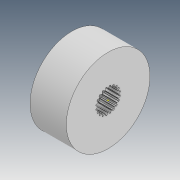
# Autodesk Inventor part: roda certa 3.0
Saved by Autodesk Inventor 2021 (Build 250183000, 183)
## iProperties
Created: 2020-10-21
Part Number: roda certa 3.0
Material: Genérico
Document SubType Name: Modeling
Designer: evert
Density: 1 g/cm^3
Appearance: Padrão
Author: evert
Autodesk Inventor part; units mm, degrees
ref_plane "YZ Plane" through (0, 0, 0) normal (1, 0, 0) x (0, 1, 0)
ref_plane "XZ Plane" through (0, 0, 0) normal (0, 1, 0) x (-1, 0, 0)
ref_plane "XY Plane" through (0, 0, 0) normal (0, 0, 1) x (1, 0, 0)
sketch "Esboço2" plane through (0, 0, 0) normal (0, 0, 1) x (1, 0, 0)
  line L0 (0, 0) -> (9.5, 0)
  line L1 (9.5, 0) -> (9.5, 9.8)
  line L2 (9.5, 9.8) -> (0, 9.8)
  line L3 (0, 9.8) -> (0, 0)
  line L4 (9.5, 0) -> (1, 0)
  line L5 (9.5, 0) -> (0.5, 0)
  line L6 (0, 0) -> (1, 0)
  line L7 (1, 0) -> (1, 9.8)
  dimension "d0" = 9.5
  dimension "d1" = 9.8
  dimension "d71" = 8.5
  dimension "d72" = 9
  constraints: 16 end point, 3 point on line, 2 parallel, 2 perpendicular, 1 collinear, 1 horizontal
  measures "d0" distance of L1.end L2.end
  measures "d1" distance of L0.end L1.end
  measures "d71" distance of L0.end L4.end
  measures "d72" distance of L0.end L5.end
revolve "Revolução1" add sketch "Esboço2" angle 360 about axis through (0, 0, 0) along (1, 0, 0) contours L7 L2 L1 L0
sketch "Esboço12" plane through (9.5, 0, 0) normal (1, 0, 0) x (0, 0, -1)
  point P0 (0, 0)
sketch "Esboço13" plane through (1, 0, 0) normal (-1, 0, 0) x (0, 0, 1)
  circle A0 centre (0, 0) radius 1.75
  dimension "d73" = 3.5
  constraints: 1 centre point, 1 coincident
  measures "d73" diameter of A0
extrude "Extrusão6" cut sketch "Esboço13" against normal blind 3.85
sketch "Esboço14" plane through (1, 0, 0) normal (-1, 0, 0) x (0, 0, 1)
  circle A0 centre (0, 0) radius 1.75 projected
  circle A1 centre (0, 0) radius 4.5
  dimension "d76" = 9
  constraints: 1 centre point, 1 coincident
  measures "d76" diameter of A1
extrude "Extrusão7" cut sketch "Esboço14" against normal blind 1
sketch "Esboço15" plane through (9.5, 0, 0) normal (1, 0, 0) x (0, 0, -1)
  circle A0 centre (0, 0) radius 2.5
  circle A1 centre (0, 0) radius 1.75 projected
  circle A2 centre (0, 0) radius 2.9
  line L0 (2.5, 0) -> (2.5, 0.05)
  line L1 (2.5, 0) -> (2.4995, -0.05)
  line L2 (2.4995, -0.05) -> (2.8824, -0.3191)
  line L3 (2.5, 0.05) -> (2.8824, 0.3191)
  line L4 (2.8824, 0.3191) -> (2.8765, 0.3688)
  line L5 (2.8824, -0.3191) -> (2.8824, -0.3191)
  line L6 (2.8824, -0.3191) -> (2.8824, -0.3191)
  line L7 (2.8824, -0.3191) -> (2.8824, -0.3191)
  line L8 (2.8824, -0.3191) -> (2.8824, -0.3191)
  line L9 (2.8824, -0.3191) -> (2.8824, -0.3191)
  line L10 (2.8795, -0.3439) -> (2.8795, -0.3439)
  line L11 (2.8824, -0.3191) -> (2.8824, -0.3191)
  line L12 (2.3622, 0.8201) -> (2.6427, 1.1942)
  line L13 (2.6427, 1.1942) -> (2.6217, 1.2396)
  line L14 (2.3776, 0.7725) -> (2.3622, 0.8201)
  line L15 (2.3776, 0.7725) -> (2.3926, 0.7248)
  line L16 (2.3926, 0.7248) -> (2.8399, 0.5872)
  circle A3 centre (0, 0) radius 2.9
  line L17 (1.9932, 1.5099) -> (2.1443, 1.9524)
  line L18 (2.1443, 1.9524) -> (2.1104, 1.9891)
  line L19 (2.0225, 1.4695) -> (1.9932, 1.5099)
  line L20 (2.0225, 1.4695) -> (2.0515, 1.4287)
  line L21 (2.0515, 1.4287) -> (2.5195, 1.4361)
  circle A4 centre (0, 0) radius 2.9
  line L22 (1.429, 2.0519) -> (1.4361, 2.5195)
  line L23 (1.4361, 2.5195) -> (1.3924, 2.5439)
  line L24 (1.4695, 2.0225) -> (1.429, 2.0519)
  line L25 (1.4695, 2.0225) -> (1.5096, 1.9928)
  line L26 (1.5096, 1.9928) -> (1.9524, 2.1443)
  circle A5 centre (0, 0) radius 2.9
  line L27 (0.725, 2.3931) -> (0.5872, 2.8399)
  line L28 (0.5872, 2.8399) -> (0.5382, 2.8496)
  line L29 (0.7725, 2.3776) -> (0.725, 2.3931)
  line L30 (0.7725, 2.3776) -> (0.8199, 2.3617)
  line L31 (0.8199, 2.3617) -> (1.1942, 2.6427)
  circle A6 centre (0, 0) radius 2.9
  line L32 (-0.05, 2.5) -> (-0.3191, 2.8824)
  line L33 (-0.3191, 2.8824) -> (-0.3688, 2.8765)
  line L34 (0, 2.5) -> (-0.05, 2.5)
  line L35 (0, 2.5) -> (0.05, 2.4995)
  line L36 (0.05, 2.4995) -> (0.3191, 2.8824)
  circle A7 centre (0, 0) radius 2.9
  line L37 (-0.8201, 2.3622) -> (-1.1942, 2.6427)
  line L38 (-1.1942, 2.6427) -> (-1.2396, 2.6217)
  line L39 (-0.7725, 2.3776) -> (-0.8201, 2.3622)
  line L40 (-0.7725, 2.3776) -> (-0.7248, 2.3926)
  line L41 (-0.7248, 2.3926) -> (-0.5872, 2.8399)
  circle A8 centre (0, 0) radius 2.9
  line L42 (-1.5099, 1.9932) -> (-1.9524, 2.1443)
  line L43 (-1.9524, 2.1443) -> (-1.9891, 2.1104)
  line L44 (-1.4695, 2.0225) -> (-1.5099, 1.9932)
  line L45 (-1.4695, 2.0225) -> (-1.4287, 2.0515)
  line L46 (-1.4287, 2.0515) -> (-1.4361, 2.5195)
  circle A9 centre (0, 0) radius 2.9
  line L47 (-2.0519, 1.429) -> (-2.5195, 1.4361)
  line L48 (-2.5195, 1.4361) -> (-2.5439, 1.3924)
  line L49 (-2.0225, 1.4695) -> (-2.0519, 1.429)
  line L50 (-2.0225, 1.4695) -> (-1.9928, 1.5096)
  line L51 (-1.9928, 1.5096) -> (-2.1443, 1.9524)
  circle A10 centre (0, 0) radius 2.9
  line L52 (-2.3931, 0.725) -> (-2.8399, 0.5872)
  line L53 (-2.8399, 0.5872) -> (-2.8496, 0.5382)
  line L54 (-2.3776, 0.7725) -> (-2.3931, 0.725)
  line L55 (-2.3776, 0.7725) -> (-2.3617, 0.8199)
  line L56 (-2.3617, 0.8199) -> (-2.6427, 1.1942)
  circle A11 centre (0, 0) radius 2.9
  line L57 (-2.5, -0.05) -> (-2.8824, -0.3191)
  line L58 (-2.8824, -0.3191) -> (-2.8765, -0.3688)
  line L59 (-2.5, 0) -> (-2.5, -0.05)
  line L60 (-2.5, 0) -> (-2.4995, 0.05)
  line L61 (-2.4995, 0.05) -> (-2.8824, 0.3191)
  circle A12 centre (0, 0) radius 2.9
  line L62 (-2.3622, -0.8201) -> (-2.6427, -1.1942)
  line L63 (-2.6427, -1.1942) -> (-2.6217, -1.2396)
  line L64 (-2.3776, -0.7725) -> (-2.3622, -0.8201)
  line L65 (-2.3776, -0.7725) -> (-2.3926, -0.7248)
  line L66 (-2.3926, -0.7248) -> (-2.8399, -0.5872)
  circle A13 centre (0, 0) radius 2.9
  line L67 (-1.9932, -1.5099) -> (-2.1443, -1.9524)
  line L68 (-2.1443, -1.9524) -> (-2.1104, -1.9891)
  line L69 (-2.0225, -1.4695) -> (-1.9932, -1.5099)
  line L70 (-2.0225, -1.4695) -> (-2.0515, -1.4287)
  line L71 (-2.0515, -1.4287) -> (-2.5195, -1.4361)
  circle A14 centre (0, 0) radius 2.9
  line L72 (-1.429, -2.0519) -> (-1.4361, -2.5195)
  line L73 (-1.4361, -2.5195) -> (-1.3924, -2.5439)
  line L74 (-1.4695, -2.0225) -> (-1.429, -2.0519)
  line L75 (-1.4695, -2.0225) -> (-1.5096, -1.9928)
  line L76 (-1.5096, -1.9928) -> (-1.9524, -2.1443)
  circle A15 centre (0, 0) radius 2.9
  line L77 (-0.725, -2.3931) -> (-0.5872, -2.8399)
  line L78 (-0.5872, -2.8399) -> (-0.5382, -2.8496)
  line L79 (-0.7725, -2.3776) -> (-0.725, -2.3931)
  line L80 (-0.7725, -2.3776) -> (-0.8199, -2.3617)
  line L81 (-0.8199, -2.3617) -> (-1.1942, -2.6427)
  circle A16 centre (0, 0) radius 2.9
  line L82 (0.05, -2.5) -> (0.3191, -2.8824)
  line L83 (0.3191, -2.8824) -> (0.3688, -2.8765)
  line L84 (0, -2.5) -> (0.05, -2.5)
  line L85 (0, -2.5) -> (-0.05, -2.4995)
  line L86 (-0.05, -2.4995) -> (-0.3191, -2.8824)
  circle A17 centre (0, 0) radius 2.9
  line L87 (0.8201, -2.3622) -> (1.1942, -2.6427)
  line L88 (1.1942, -2.6427) -> (1.2396, -2.6217)
  line L89 (0.7725, -2.3776) -> (0.8201, -2.3622)
  line L90 (0.7725, -2.3776) -> (0.7248, -2.3926)
  line L91 (0.7248, -2.3926) -> (0.5872, -2.8399)
  circle A18 centre (0, 0) radius 2.9
  line L92 (1.5099, -1.9932) -> (1.9524, -2.1443)
  line L93 (1.9524, -2.1443) -> (1.9891, -2.1104)
  line L94 (1.4695, -2.0225) -> (1.5099, -1.9932)
  line L95 (1.4695, -2.0225) -> (1.4287, -2.0515)
  line L96 (1.4287, -2.0515) -> (1.4361, -2.5195)
  circle A19 centre (0, 0) radius 2.9
  line L97 (2.0519, -1.429) -> (2.5195, -1.4361)
  line L98 (2.5195, -1.4361) -> (2.5439, -1.3924)
  line L99 (2.0225, -1.4695) -> (2.0519, -1.429)
  line L100 (2.0225, -1.4695) -> (1.9928, -1.5096)
  line L101 (1.9928, -1.5096) -> (2.1443, -1.9524)
  circle A20 centre (0, 0) radius 2.9
  line L102 (2.3931, -0.725) -> (2.8399, -0.5872)
  line L103 (2.8399, -0.5872) -> (2.8496, -0.5382)
  line L104 (2.3776, -0.7725) -> (2.3931, -0.725)
  line L105 (2.3776, -0.7725) -> (2.3617, -0.8199)
  line L106 (2.3617, -0.8199) -> (2.6427, -1.1942)
  circle A21 centre (0, 0) radius 2.9
  point P0 (2.8399, 0.5872)
  point P1 (2.8399, 0.5872)
  point P2 (2.8399, 0.5872)
  point P3 (2.8399, 0.5872)
  point P4 (2.8399, 0.5872)
  point P5 (2.8449, 0.5627)
  point P6 (2.8449, 0.5627)
  point P7 (2.8399, 0.5872)
  point P8 (2.5195, 1.4361)
  point P9 (2.5195, 1.4361)
  point P10 (2.5195, 1.4361)
  point P11 (2.5195, 1.4361)
  point P12 (2.5195, 1.4361)
  point P13 (2.5318, 1.4143)
  point P14 (2.5318, 1.4143)
  point P15 (2.5195, 1.4361)
  point P16 (1.9524, 2.1443)
  point P17 (1.9524, 2.1443)
  point P18 (1.9524, 2.1443)
  point P19 (1.9524, 2.1443)
  point P20 (1.9524, 2.1443)
  point P21 (1.9708, 2.1274)
  point P22 (1.9708, 2.1274)
  point P23 (1.9524, 2.1443)
  point P24 (1.1942, 2.6427)
  point P25 (1.1942, 2.6427)
  point P26 (1.1942, 2.6427)
  point P27 (1.1942, 2.6427)
  point P28 (1.1942, 2.6427)
  point P29 (1.2169, 2.6323)
  point P30 (1.2169, 2.6323)
  point P31 (1.1942, 2.6427)
  point P32 (0.3191, 2.8824)
  point P33 (0.3191, 2.8824)
  point P34 (0.3191, 2.8824)
  point P35 (0.3191, 2.8824)
  point P36 (0.3191, 2.8824)
  point P37 (0.3439, 2.8795)
  point P38 (0.3439, 2.8795)
  point P39 (0.3191, 2.8824)
  point P40 (-0.5872, 2.8399)
  point P41 (-0.5872, 2.8399)
  point P42 (-0.5872, 2.8399)
  point P43 (-0.5872, 2.8399)
  point P44 (-0.5872, 2.8399)
  point P45 (-0.5627, 2.8449)
  point P46 (-0.5627, 2.8449)
  point P47 (-0.5872, 2.8399)
  point P48 (-1.4361, 2.5195)
  point P49 (-1.4361, 2.5195)
  point P50 (-1.4361, 2.5195)
  point P51 (-1.4361, 2.5195)
  point P52 (-1.4361, 2.5195)
  point P53 (-1.4143, 2.5318)
  point P54 (-1.4143, 2.5318)
  point P55 (-1.4361, 2.5195)
  point P56 (-2.1443, 1.9524)
  point P57 (-2.1443, 1.9524)
  point P58 (-2.1443, 1.9524)
  point P59 (-2.1443, 1.9524)
  point P60 (-2.1443, 1.9524)
  point P61 (-2.1274, 1.9708)
  point P62 (-2.1274, 1.9708)
  point P63 (-2.1443, 1.9524)
  point P64 (-2.6427, 1.1942)
  point P65 (-2.6427, 1.1942)
  point P66 (-2.6427, 1.1942)
  point P67 (-2.6427, 1.1942)
  point P68 (-2.6427, 1.1942)
  point P69 (-2.6323, 1.2169)
  point P70 (-2.6323, 1.2169)
  point P71 (-2.6427, 1.1942)
  point P72 (-2.8824, 0.3191)
  point P73 (-2.8824, 0.3191)
  point P74 (-2.8824, 0.3191)
  point P75 (-2.8824, 0.3191)
  point P76 (-2.8824, 0.3191)
  point P77 (-2.8795, 0.3439)
  point P78 (-2.8795, 0.3439)
  point P79 (-2.8824, 0.3191)
  point P80 (-2.8399, -0.5872)
  point P81 (-2.8399, -0.5872)
  point P82 (-2.8399, -0.5872)
  point P83 (-2.8399, -0.5872)
  point P84 (-2.8399, -0.5872)
  point P85 (-2.8449, -0.5627)
  point P86 (-2.8449, -0.5627)
  point P87 (-2.8399, -0.5872)
  point P88 (-2.5195, -1.4361)
  point P89 (-2.5195, -1.4361)
  point P90 (-2.5195, -1.4361)
  point P91 (-2.5195, -1.4361)
  point P92 (-2.5195, -1.4361)
  point P93 (-2.5318, -1.4143)
  point P94 (-2.5318, -1.4143)
  point P95 (-2.5195, -1.4361)
  point P96 (-1.9524, -2.1443)
  point P97 (-1.9524, -2.1443)
  point P98 (-1.9524, -2.1443)
  point P99 (-1.9524, -2.1443)
  point P100 (-1.9524, -2.1443)
  point P101 (-1.9708, -2.1274)
  point P102 (-1.9708, -2.1274)
  point P103 (-1.9524, -2.1443)
  point P104 (-1.1942, -2.6427)
  point P105 (-1.1942, -2.6427)
  point P106 (-1.1942, -2.6427)
  point P107 (-1.1942, -2.6427)
  point P108 (-1.1942, -2.6427)
  point P109 (-1.2169, -2.6323)
  point P110 (-1.2169, -2.6323)
  point P111 (-1.1942, -2.6427)
  point P112 (-0.3191, -2.8824)
  point P113 (-0.3191, -2.8824)
  point P114 (-0.3191, -2.8824)
  point P115 (-0.3191, -2.8824)
  point P116 (-0.3191, -2.8824)
  point P117 (-0.3439, -2.8795)
  point P118 (-0.3439, -2.8795)
  point P119 (-0.3191, -2.8824)
  point P120 (0.5872, -2.8399)
  point P121 (0.5872, -2.8399)
  point P122 (0.5872, -2.8399)
  point P123 (0.5872, -2.8399)
  point P124 (0.5872, -2.8399)
  point P125 (0.5627, -2.8449)
  point P126 (0.5627, -2.8449)
  point P127 (0.5872, -2.8399)
  point P128 (1.4361, -2.5195)
  point P129 (1.4361, -2.5195)
  point P130 (1.4361, -2.5195)
  point P131 (1.4361, -2.5195)
  point P132 (1.4361, -2.5195)
  point P133 (1.4143, -2.5318)
  point P134 (1.4143, -2.5318)
  point P135 (1.4361, -2.5195)
  point P136 (2.1443, -1.9524)
  point P137 (2.1443, -1.9524)
  point P138 (2.1443, -1.9524)
  point P139 (2.1443, -1.9524)
  point P140 (2.1443, -1.9524)
  point P141 (2.1274, -1.9708)
  point P142 (2.1274, -1.9708)
  point P143 (2.1443, -1.9524)
  point P144 (2.6427, -1.1942)
  point P145 (2.6427, -1.1942)
  point P146 (2.6427, -1.1942)
  point P147 (2.6427, -1.1942)
  point P148 (2.6427, -1.1942)
  point P149 (2.6323, -1.2169)
  point P150 (2.6323, -1.2169)
  point P151 (2.6427, -1.1942)
  dimension "d79" = 5
  dimension "d80" = 5.8
  dimension "d81" = 0.05
  dimension "d82" = 0.05
  dimension "d83" = 0.468
  dimension "d85" = 0.05
  dimension "d88" = 360
  constraints: 214 end point, 2 coincident, 2 vertical, 692 other
  measures "d81" distance of L0.start L0.end
  measures "d82" distance of L0.start L1.end
  measures "d83" distance of L1.end L2.end
  measures "d85" distance of L3.end L4.end
extrude "Extrusão8" cut sketch "Esboço15" against normal blind 3.5 contours A0 | A0 L16 A2 L3 | L2 A2 L102 A0 | A0 L21 A2 L12 | L106 A2 L97 A0 | A0 L26 A2 L17 | L101 A2 L92 A0 | A0 L31 A2 L22 | L96 A2 L87 A0 | A0 L36 A2 L27 | L91 A2 L82 A0 | A0 L41 A2 L32 | L86 A2 L77 A0 | A0 L46 A2 L37 | L81 A2 L72 A0 | A0 L51 A2 L42 | L76 A2 L67 A0 | A0 L56 A2 L47 | L71 A2 L62 A0 | A0 L61 A2 L52 | L66 A2 L57 A0 | A1
